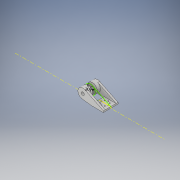
# Autodesk Inventor part: bridge3
Saved by Autodesk Inventor 2019 (Build 230136000, 136)
## iProperties
Created: 2019-02-10
Part Number: bridge3
Material: Generic
Document SubType Name: Modeling
Designer: BOXI
Density: 1 g/cm^3
Appearance: Default
Author: BOXI
Autodesk Inventor part; units mm, degrees
ref_plane "YZ Plane" through (0, 0, 0) normal (1, 0, 0) x (0, 1, 0)
ref_plane "XZ Plane" through (0, 0, 0) normal (0, 1, 0) x (-1, 0, 0)
ref_plane "XY Plane" through (0, 0, 0) normal (0, 0, 1) x (1, 0, 0)
sketch "Sketch2" plane through (0, 0, 0) normal (0, 0, 1) x (1, 0, 0)
  line L0 (-16.8, 0) -> (16.8, 0) construction
  line L1 (0, -21) -> (0, 21) construction
  line L2 (-12, -15) -> (12, -15)
  line L3 (12, -15) -> (12, 15)
  line L4 (12, 15) -> (-12, 15)
  line L5 (-12, 15) -> (-12, -15)
  circle A0 centre (7.02, 0) radius 1
  circle A1 centre (4.96389, 4.96389) radius 1
  circle A2 centre (0, 7.02) radius 1
  circle A3 centre (-4.96389, 4.96389) radius 1
  circle A4 centre (-7.02, 0) radius 1
  circle A5 centre (-4.96389, -4.96389) radius 1
  circle A6 centre (0, -7.02) radius 1
  circle A7 centre (4.96389, -4.96389) radius 1
  point P0 (0, 0)
  dimension "d3" = 30
  dimension "d4" = 24
  dimension "d5" = 7.02
  dimension "d6" = 2
  dimension "d9" = 360
  constraints: 8 centre point, 8 end point, 2 parallel, 1 horizontal, 1 perpendicular, 1 point on line, 19 other
  measures "d3" distance of L2.end L3.end
  measures "d4" distance of L3.end L4.end
  measures "d5" distance of point (0, 0) A0.centre
  measures "d6" diameter of A0
extrude "Extrusion1" add sketch "Sketch2" along normal blind 3 contours L5 L4 L3 L2 | A0 | A1 | A2 | A3 | A4 | A5 | A6 | A7
sketch "Sketch1" plane through (0, 0, 0) normal (0, 1, 0) x (-1, 0, 0)
  line L0 (183.866798, 0) -> (-123.200788, 0) construction
  line L1 (-12, 0) -> (12, 0)
  line L2 (12, 0) -> (12, 3)
  line L3 (-12, 3) -> (12, 3)
  line L4 (-12, 0) -> (-12, 3)
  circle A0 centre (30, 12.361524) radius 10
  line L5 (-12, 0) -> (-12, 3)
  line L6 (25.615753, 21.349203) -> (-12, 3)
  line L7 (31.257448, 2.440898) -> (12, 0)
  circle A1 centre (30, 12.361524) radius 3
  dimension "d31" = 20
  dimension "d32" = 6
  constraints: 4 end point, 2 centre point, 2 point on circle, 2 tangent, 1 coincident
  measures "d31" diameter of A0
  measures "d32" diameter of A1
extrude "Extrusion6" add sketch "Sketch1" along normal blind 4 from surface at -15 contours L2 L3 L6 A0 L7 | A0 | A1
mirror "Mirror1" about plane through (0, 0, 0) normal (0, 1, 0) of "Extrusion6"
extrude "Extrusion7" cut sketch "Sketch2" along normal through all contours A0 | A1 | A2 | A3 | A4 | A5 | A6 | A7
extrude "Extrusion8" add sketch "Sketch1" along normal through all both and the other way through all contours A0 | A1
extrude "Extrusion9" cut sketch "Sketch1" along normal mid plane 9 contours A0 | A1
extrude "Extrusion10" cut sketch "Sketch1" along normal through all both and the other way through all contours A1
body "Solid1"
